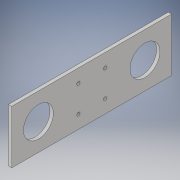
# Autodesk Inventor part: 2AM-17-P-0206  - slider plate
Saved by Autodesk Inventor 2017 (Build 210142000, 142)
## iProperties
Created: 2017-12-27
Part Number: 2AM-17-P-0206  - slider plate
Material: Generic
Document SubType Name: Modeling
Designer: Micah
Density: 1 g/cm^3
Appearance: Default
Author: Micah
Autodesk Inventor part; units mm, degrees
ref_plane "YZ Plane" through (0, 0, 0) normal (1, 0, 0) x (0, 1, 0)
ref_plane "XZ Plane" through (0, 0, 0) normal (0, 1, 0) x (-1, 0, 0)
ref_plane "XY Plane" through (0, 0, 0) normal (0, 0, 1) x (1, 0, 0)
sketch "Sketch1" plane through (0, 0, 0) normal (1, 0, 0) x (0, 1, 0)
  line L0 (0, 0) -> (50.8, 0)
  line L1 (50.8, 0) -> (50.8, 152.4)
  line L2 (50.8, 152.4) -> (0, 152.4)
  line L3 (0, 152.4) -> (0, 0)
  line L4 (50.8, 0) -> (50.8, 25.4) construction
  line L5 (50.8, 25.4) -> (0, 25.4) construction
  line L6 (25.4, 0) -> (25.4, 25.4) construction
  circle A0 centre (25.4, 25.4) radius 14.2875
  line L7 (50.8, 25.4) -> (50.8, 38.1) construction
  line L8 (50.8, 76.2) -> (0, 76.2) construction
  circle A1 centre (25.4, 127) radius 14.2875
  line L9 (50.8, 76.2) -> (50.8, 88.9) construction
  line L10 (50.8, 88.9) -> (38.1, 88.9) construction
  circle A2 centre (38.1, 88.9) radius 1.5875
  line L11 (25.4, 152.4) -> (25.4, 0) construction
  circle A3 centre (38.1, 63.5) radius 1.5875
  circle A4 centre (12.7, 88.9) radius 1.5875
  circle A5 centre (12.7, 63.5) radius 1.5875
  dimension "d11" = 50.8
  dimension "d12" = 152.4
  dimension "d13" = 25.4
  dimension "d14" = 28.575
  dimension "d22" = 12.7
  dimension "d23" = 12.7
  dimension "d24" = 3.175
  constraints: 24 end point, 6 centre point, 5 midpoint, 4 point on line, 4 symmetric about line, 3 perpendicular, 2 coincident, 2 parallel, 1 collinear, 1 horizontal, 4 other
  measures "d11" distance of L2.end L1.end
  measures "d12" distance of L1.end L0.end
  measures "d13" distance of L0.end L4.end
  measures "d14" diameter of A0
  measures "d22" distance of L8.start L9.end
  measures "d23" distance of L9.end L10.end
  measures "d24" diameter of A2
extrude "Extrusion2" add sketch "Sketch1" along normal blind 3.175
body "Solid2"
